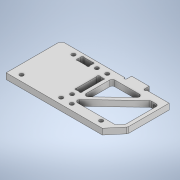
# Autodesk Inventor part: Trunk_lower_side_frame
Saved by Autodesk Inventor 2020.4 (Build 244396000, 396)
## iProperties
Created: 2022-01-02
Part Number: Trunk_lower_side_frame
Material: 一般
Document SubType Name: Modeling
Designer: Masato Kubotera
Density: 1 g/cm^3
Appearance: 既定
Author: Masato Kubotera
Autodesk Inventor part; units mm, degrees
ref_plane "YZ Plane" through (0, 0, 0) normal (1, 0, 0) x (0, 1, 0)
ref_plane "XZ Plane" through (0, 0, 0) normal (0, 1, 0) x (-1, 0, 0)
ref_plane "XY Plane" through (0, 0, 0) normal (0, 0, 1) x (1, 0, 0)
derived "Trunk_basis.ipt"
sketch "スケッチ1" plane through (0, 0, 0) normal (0, 1, 0) x (-1, 0, 0)
  line L0 (0, 22) -> (0, -139) construction
  circle A0 centre (5, 0) radius 10.5 construction
  line L1 (-7, 16) -> (36, 16) construction
  line L2 (36, 16) -> (36, -16) construction
  line L3 (36, -16) -> (-7, -16) construction
  line L4 (-7, -16) -> (-7, 16) construction
  line L5 (-7, 16) -> (36, -16) construction
  line L6 (36, 16) -> (-7, -16) construction
  line L7 (33, 13.5) -> (6, 13.5) construction
  line L8 (6, 13.5) -> (6, -13.5) construction
  line L9 (6, -13.5) -> (33, -13.5) construction
  line L10 (33, -13.5) -> (33, 13.5) construction
  line L11 (33, 13.5) -> (6, -13.5) construction
  line L12 (6, 13.5) -> (33, -13.5) construction
  line L13 (-7, 0) -> (36, 0) construction
  arc A1 (5, 16) -> (-7, 10.583) centre (5, 0) ccw construction
  line L14 (34.5651, -16.05) -> (5, -16.05)
  line L15 (5, 16.05) -> (34.5651, 16.05)
  line L16 (36.05, 14.5651) -> (36.05, -14.5651)
  line L17 (36.05, -16.05) -> (-7.05, 16.05) construction
  line L18 (-7.05, -16.05) -> (36.05, 16.05) construction
  arc A2 (5, 16.05) -> (-6.5314, 11.1638) centre (5, 0) ccw
  arc A3 (-6.5314, 11.1638) -> (-7.05, 9.8372) centre (-6.0721, 10.2196) ccw
  arc A4 (36.05, 14.5651) -> (34.5651, 16.05) centre (35.3075, 15.3075) ccw
  circle A5 centre (6, 13.5) radius 1.35 construction
  line L19 (19.5, 13.5) -> (19.5, -13.5) construction
  circle A6 centre (33, 13.5) radius 1.35 construction
  line L20 (-12, 22) -> (-14.5, 19.5)
  line L21 (-14.5, 19.5) -> (-14.5, -13.5)
  line L22 (-14.5, -13.5) -> (-28.5, -27.5)
  line L23 (-28.5, -27.5) -> (-28.5, -94.5)
  line L24 (91.5, -94.5) -> (91.5, -22.5)
  line L25 (91.5, -22.5) -> (52, 0.3053)
  line L26 (52, 0.3053) -> (52, 19.5)
  line L27 (52, 19.5) -> (49.5, 22)
  line L28 (49.5, 22) -> (-12, 22)
  line L29 (-18.5, -92) -> (-28.5, -103.8625)
  line L30 (-28.5, -103.8625) -> (-28.5, -139)
  line L31 (-28.5, -139) -> (63.5, -139)
  line L32 (63.5, -139) -> (63.5, -92)
  line L33 (63.5, -92) -> (-18.5, -92)
  line L34 (-16, -139) -> (-16, -99.5) construction
  line L35 (-16, -99.5) -> (16, -99.5) construction
  line L36 (16, -139) -> (16, -99.5) construction
  line L37 (-7.5, -139) -> (-7.5, -143)
  line L38 (-7.5, -143) -> (7.5, -143)
  line L39 (7.5, -139) -> (7.5, -143)
  arc A7 (-7.5, -139) -> (-9.6, -139) centre (-8.55, -139) ccw
  arc A8 (9.6, -139) -> (7.5, -139) centre (8.55, -139) ccw
  line L40 (-22, -139) -> (-22, -133) construction
  line L41 (-23.5, -133) -> (-20.5, -133) construction
  line L42 (-23.5, -133) -> (-23.5, -139) construction
  line L43 (-20.5, -133) -> (-20.5, -139) construction
  line L44 (-12, 22) -> (-7, 22) construction
  line L45 (-7, 22) -> (-7, -22) construction
  line L46 (-7, -22) -> (-12, -22) construction
  line L47 (-12, -22) -> (-12, 22) construction
  line L48 (-12, 22) -> (-7, -22) construction
  line L49 (-7, 22) -> (-12, -22) construction
  line L50 (-9.5, 22) -> (-9.5, -22) construction
  line L51 (-7, 0) -> (-12, 0) construction
  circle A9 centre (-9.5, 17.75) radius 1.6
  line L52 (-12, 10) -> (-9.5, 10) construction
  line L53 (-9.5, 10) -> (-9.5, -10) construction
  line L54 (-9.5, -10) -> (-12, -10) construction
  line L55 (-12, -10) -> (-12, 10) construction
  line L56 (-12, 10) -> (-9.5, -10) construction
  line L57 (-9.5, 10) -> (-12, -10) construction
  line L58 (-9.45, 10.05) -> (-12.05, 10.05)
  line L59 (-12.05, 7.95) -> (-12.05, -7.95)
  line L60 (-12.05, -10.05) -> (-9.45, -10.05)
  line L61 (-9.45, -7.95) -> (-9.45, 7.95)
  line L62 (-9.45, 10.05) -> (-12.05, -10.05) construction
  line L63 (-12.05, 10.05) -> (-9.45, -10.05) construction
  arc A10 (-12.05, 10.05) -> (-12.05, 7.95) centre (-12.05, 9) ccw
  line L64 (-10.75, 10) -> (-10.75, -10) construction
  arc A11 (-9.45, 7.95) -> (-9.45, 10.05) centre (-9.45, 9) ccw
  circle A12 centre (-9.5, -17.75) radius 1.6
  arc A13 (-12.05, -7.95) -> (-12.05, -10.05) centre (-12.05, -9) ccw
  arc A14 (-9.45, -10.05) -> (-9.45, -7.95) centre (-9.45, -9) ccw
  line L65 (36, 14.4) -> (44.5, 14.4) construction
  line L66 (44.5, 14.4) -> (44.5, -14.4) construction
  line L67 (36, -14.4) -> (44.5, -14.4) construction
  line L68 (46.95, 7.95) -> (46.95, -7.95)
  line L69 (49.5, 0) -> (44.5, 0) construction
  line L70 (44.5, 22) -> (49.5, 22) construction
  line L71 (49.55, -7.95) -> (49.55, 7.95)
  line L72 (48.25, 10) -> (48.25, -10) construction
  line L73 (49.5, 10) -> (47, -10) construction
  line L74 (49.5, -10) -> (47, -10) construction
  line L75 (49.5, 10) -> (49.5, -10) construction
  line L76 (47, 10) -> (49.5, -10) construction
  line L77 (46.95, -10.05) -> (49.55, -10.05)
  line L78 (46.95, 10.05) -> (49.55, -10.05) construction
  line L79 (49.55, 10.05) -> (46.95, -10.05) construction
  line L80 (49.5, -22) -> (44.5, -22) construction
  line L81 (44.5, 22) -> (49.5, -22) construction
  line L82 (49.5, 22) -> (49.5, -22) construction
  line L83 (49.5, 22) -> (44.5, -22) construction
  line L84 (47, 22) -> (47, -22) construction
  line L85 (44.5, -22) -> (44.5, 22) construction
  circle A15 centre (47, -17.75) radius 1.6
  arc A16 (49.55, -10.05) -> (49.55, -7.95) centre (49.55, -9) ccw
  line L86 (47, -10) -> (47, 10) construction
  arc A17 (46.95, -7.95) -> (46.95, -10.05) centre (46.95, -9) ccw
  arc A18 (46.95, 10.05) -> (46.95, 7.95) centre (46.95, 9) ccw
  arc A19 (49.55, 7.95) -> (49.55, 10.05) centre (49.55, 9) ccw
  line L87 (47, 10) -> (49.5, 10) construction
  line L88 (49.55, 10.05) -> (46.95, 10.05)
  circle A20 centre (47, 17.75) radius 1.6
  line L89 (-18.5, -99.5) -> (-28.5, -94.5)
  line L90 (-18.5, -99.5) -> (63.5, -99.5)
  circle A21 centre (55.4106, -97) radius 1.6
  line L91 (21.0546, -94.5) -> (56, -94.5) construction
  line L92 (56, -94.5) -> (56, -99.5) construction
  line L93 (56, -99.5) -> (21.0546, -99.5) construction
  line L94 (21.0546, -99.5) -> (21.0546, -94.5) construction
  line L95 (21.0546, -94.5) -> (56, -99.5) construction
  line L96 (56, -94.5) -> (21.0546, -99.5) construction
  line L97 (21.0546, -97) -> (56, -97) construction
  line L98 (-18.5, -92) -> (-18.5, -99.5) construction
  line L99 (38.5273, -99.5) -> (38.5273, -94.5) construction
  circle A22 centre (21.644, -97) radius 1.6
  line L100 (-28.5, -94.5) -> (91.5, -94.5) construction
  line L101 (91.5, -94.5) -> (63.5, -99.5)
  circle A23 centre (5, 0) radius 16 construction
  arc A24 (-6.5314, -11.1638) -> (5, -16.05) centre (5, 0) ccw
  arc A25 (-7.05, -9.8372) -> (-6.5314, -11.1638) centre (-6.0721, -10.2196) ccw
  arc A26 (34.5651, -16.05) -> (36.05, -14.5651) centre (35.3075, -15.3075) ccw
  line L102 (-7.05, -9.8372) -> (-7.05, 9.8372)
  line L103 (22, -139) -> (22, -133) construction
  line L104 (23.5, -133) -> (23.5, -139) construction
  line L105 (20.5, -133) -> (20.5, -139) construction
  line L106 (23.5, -133) -> (20.5, -133) construction
  circle A27 centre (6, -13.5) radius 1.35
  circle A28 centre (33, -13.5) radius 1.35
  line L107 (61, -139) -> (63.5, -136.5)
  line L108 (61, -94.5) -> (56, -94.5)
  line L109 (56, -94.5) -> (56, -139) construction
  line L110 (56, -139) -> (61, -139) construction
  line L111 (61, -139) -> (61, -94.5)
  line L112 (61, -94.5) -> (56, -139) construction
  line L113 (56, -94.5) -> (61, -139) construction
  line L114 (22, -108.5) -> (56, -108.5) construction
  line L115 (56, -108.5) -> (56, -131.5) construction
  line L116 (56, -131.5) -> (22, -131.5) construction
  line L117 (22, -131.5) -> (22, -108.5) construction
  line L118 (22, -108.5) -> (56, -131.5) construction
  line L119 (56, -108.5) -> (22, -131.5) construction
  line L120 (22, -131.5) -> (54.2213, -131.5) construction
  line L121 (54.2213, -131.5) -> (54.2213, -136.5) construction
  line L122 (54.2213, -136.5) -> (22, -136.5) construction
  line L123 (22, -136.5) -> (22, -131.5) construction
  line L124 (22, -131.5) -> (54.2213, -136.5) construction
  line L125 (54.2213, -131.5) -> (22, -136.5) construction
  line L126 (-25.5, -133) -> (-25.5, -104.9583)
  line L127 (-21.4417, -100.1441) -> (14, -100.1441)
  line L128 (-14.1608, -133) -> (14, -133)
  line L129 (14, -133) -> (14, -106.0524)
  line L130 (14, -106.0524) -> (-14.1608, -133)
  line L131 (22, -99.5) -> (17, -99.5) construction
  line L132 (17, -99.5) -> (17, -139) construction
  line L133 (17, -139) -> (22, -139) construction
  line L134 (22, -139) -> (22, -99.5) construction
  line L135 (22, -99.5) -> (17, -139) construction
  line L136 (17, -99.5) -> (22, -139) construction
  line L137 (19.5, -99.5) -> (19.5, -139) construction
  circle A29 centre (19.5, -104.25) radius 1.6
  line L138 (17, -119.25) -> (22, -119.25) construction
  line L139 (-28.5, -139) -> (-28.5, -143) construction
  line L140 (-28.5, -143) -> (-7.5, -143) construction
  line L141 (28.5, -143) -> (7.5, -143) construction
  line L142 (28.5, -139) -> (28.5, -143) construction
  circle A30 centre (19.5, -134.25) radius 1.6
  line L143 (17, -109.25) -> (22, -109.25) construction
  line L144 (17, -129.25) -> (22, -129.25) construction
  line L145 (39.4409, -150.6176) -> (61.7571, -150.6176)
  line L146 (63.242, -152.1025) -> (63.242, -179.9354)
  line L147 (61.7571, -181.4204) -> (39.4409, -181.4204)
  line L148 (37.9559, -179.9354) -> (37.9559, -152.1025)
  line L149 (37.9559, -150.6176) -> (63.242, -181.4204) construction
  line L150 (63.242, -150.6176) -> (37.9559, -181.4204) construction
  arc A31 (39.4409, -150.6176) -> (37.9559, -152.1025) centre (38.6984, -151.36) ccw
  line L151 (50.599, -150.6176) -> (50.599, -181.4204) construction
  line L152 (37.9559, -166.019) -> (63.242, -166.019) construction
  arc A32 (63.242, -152.1025) -> (61.7571, -150.6176) centre (62.4995, -151.36) ccw
  arc A33 (37.9559, -179.9354) -> (39.4409, -181.4204) centre (38.6984, -180.6779) ccw
  arc A34 (61.7571, -181.4204) -> (63.242, -179.9354) centre (62.4995, -180.6779) ccw
  arc A35 (18.4349, -109.2) -> (16.95, -110.6849) centre (17.6925, -109.9425) ccw
  line L153 (18.4349, -109.2) -> (20.5651, -109.2)
  arc A36 (22.05, -110.6849) -> (20.5651, -109.2) centre (21.3075, -109.9425) ccw
  line L154 (16.95, -127.8151) -> (16.95, -110.6849)
  line L155 (16.95, -119.25) -> (22.05, -119.25) construction
  arc A37 (16.95, -127.8151) -> (18.4349, -129.3) centre (17.6925, -128.5575) ccw
  line L156 (19.5, -109.2) -> (19.5, -129.3) construction
  line L157 (16.95, -109.2) -> (22.05, -129.3) construction
  line L158 (22.05, -109.2) -> (16.95, -129.3) construction
  line L159 (20.5651, -129.3) -> (18.4349, -129.3)
  line L160 (22.05, -110.6849) -> (22.05, -127.8151)
  arc A38 (20.5651, -129.3) -> (22.05, -127.8151) centre (21.3075, -128.5575) ccw
  line L161 (38.1107, -131.5) -> (38.1107, -136.5) construction
  line L162 (33.1107, -131.5) -> (33.1107, -136.5) construction
  line L163 (54.2213, -134) -> (22, -134)
  circle A39 centre (28.1107, -134) radius 1.6
  arc A40 (43.1607, -132.9349) -> (41.6757, -131.45) centre (42.4182, -132.1925) ccw
  arc A41 (34.5456, -131.45) -> (33.0607, -132.9349) centre (33.8031, -132.1925) ccw
  line L164 (33.0607, -134) -> (43.1607, -134) construction
  line L165 (34.5456, -131.45) -> (41.6757, -131.45)
  line L166 (43.1607, -132.9349) -> (43.1607, -135.0651)
  line L167 (41.6757, -136.55) -> (34.5456, -136.55)
  line L168 (33.0607, -135.0651) -> (33.0607, -132.9349)
  line L169 (33.0607, -131.45) -> (43.1607, -136.55) construction
  line L170 (43.1607, -131.45) -> (33.0607, -136.55) construction
  line L171 (38.1107, -131.45) -> (38.1107, -136.55) construction
  arc A42 (33.0607, -135.0651) -> (34.5456, -136.55) centre (33.8031, -135.8075) ccw
  arc A43 (41.6757, -136.55) -> (43.1607, -135.0651) centre (42.4182, -135.8075) ccw
  line L172 (43.1107, -131.5) -> (43.1107, -136.5) construction
  circle A44 centre (48.1107, -134) radius 1.6
  circle A45 centre (-12.5, -97) radius 1.6
  circle A46 centre (12.5, -97) radius 1.6
  line L173 (-21.4417, -100.1441) -> (-25.5, -104.9583)
  line L174 (-25.5, -133) -> (-18.5, -133)
  line L175 (-18.5, -133) -> (14, -101.9001)
  line L176 (14, -101.9001) -> (14, -100.1441)
  line L177 (-23.5, -22.5) -> (91.5, -22.5) construction
  point P0 (0, 0)
  point P1 (14.5, 0)
  point P2 (19.5, 0)
  point P3 (-7.05, 10.6019)
  point P4 (19.5, 0)
  point P5 (-9.5, 0)
  point P6 (-10.75, 0)
  point P7 (36.05, 14.4)
  point P8 (36.05, -14.4)
  point P9 (48.25, 0)
  point P10 (47, 0)
  point P11 (38.5273, -97)
  point P12 (58.5, -116.75)
  point P13 (39, -120)
  point P14 (38.1107, -134)
  point P15 (19.5, -119.25)
  point P16 (50.599, -166.019)
  point P17 (19.5, -119.25)
  point P18 (19.5, -119.25)
  point P19 (38.1107, -134)
  point P20 (38.1107, -134)
  dimension "d4" = 44
  measures "d4" distance of L103.start L40.start
extrude "押し出し1" add sketch "スケッチ1" along normal blind 5 contours L89 L90 L111 L31 A8 A7 L30 L29 | L29 L33 L32 L90 L89 | L32 L107 L111 L90 | L31 L39 L38 L37
sketch "スケッチ2" plane through (28.5, 0, -139) normal (0, 0, -1) x (-1, 0, 0)
  line L0 (0, 0) -> (0, 5) projected
  line L1 (0, 2.5) -> (104.939, 2.5)
  line L2 (28.5, 0) -> (28.5, 5)
  line L3 (21, 5) -> (36, 5) projected
  point P0 (6.5, 2.5)
  point P1 (50.5, 2.5)
  dimension "d3" = 44
  constraints: 4 end point, 2 midpoint, 1 point on line, 1 symmetric about line, 1 vertical
  measures "d3" distance of point (50.5, 2.5) point (6.5, 2.5)
hole "穴1" at (22, 2.5, -139) at (-22, 2.5, -139) direction (0, 0, 1) diameter 2.459 depth 6 tip angle 118 thread size "M3x0.5" class "6H" standard "ISO Metric profile"
fillet "フィレット1" radius 2 10 edges at (25.5, 2.5, -133) (18.5, 2.5, -133) (14.1608, 2.5, -133) (-14, 2.5, -133) (-14, 2.5, -106.0524) (-14, 2.5, -100.1441) (-14, 2.5, -101.9001) (21.4417, 2.5, -100.1441) (25.5, 2.5, -104.9583) (28.5, 2.5, -103.8625)
equation "\"d3\" = d4"
